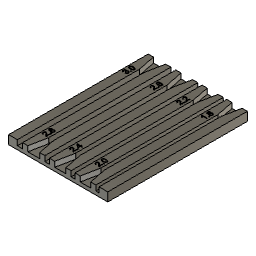
test_grooves (Autodesk Fusion 360 design; units mm, degrees)
Autodesk Fusion 360 part; units mm, degrees
sketch "Sketch1" plane through (0, 0, 0) normal (0, 0, 1) x (1, 0, 0)
  line L0 (0, 0) -> (56.8, 0)
  line L1 (56.8, 80) -> (0, 80)
  line L2 (0, 80) -> (0, 0)
  line L3 (0, 70) -> (117.6, 70) construction
  line L4 (5, 70) -> (5, 0)
  line L5 (8, 0) -> (8, 70)
  line L6 (5, 70) -> (3, 80)
  line L7 (8, 70) -> (10, 80)
  line L8 (20.8, 0) -> (20.8, 70)
  line L9 (23.4, 0) -> (23.4, 70)
  line L10 (35.8, 70) -> (35.8, 0)
  line L11 (38, 0) -> (38, 70)
  line L12 (18.8, 80) -> (20.8, 70)
  line L13 (25.4, 80) -> (23.4, 70)
  line L14 (50, 70) -> (50, 0)
  line L15 (51.8, 0) -> (51.8, 70)
  line L16 (35.8, 70) -> (33.8, 80)
  line L17 (38, 70) -> (40, 80)
  line L18 (50, 70) -> (48, 80)
  line L19 (51.8, 70) -> (53.8, 80)
  line L20 (56.8, 80) -> (56.8, 0)
  line L21 (0, 10) -> (56.8, 10) construction
  line L22 (13, 10) -> (13, 80)
  line L23 (15.8, 10) -> (15.8, 80)
  line L24 (13, 10) -> (11, 0)
  line L25 (15.8, 10) -> (17.8, 0)
  line L26 (28.4, 10) -> (28.4, 80)
  line L27 (30.8, 10) -> (30.8, 80)
  line L28 (43, 10) -> (43, 80)
  line L29 (45, 10) -> (45, 80)
  line L30 (28.4, 10) -> (26.4, 0)
  line L31 (30.8, 10) -> (32.8, 0)
  line L32 (43, 10) -> (41, 0)
  line L33 (45, 10) -> (47, 0)
  line L34 (4.6901, 63.9511) -> (4.6901, 69.9511) construction
  line L35 (4.6901, 69.9511) -> (0.6901, 69.9511) construction
  line L36 (0.6901, 69.9511) -> (0.6901, 63.9511) construction
  line L37 (0.6901, 63.9511) -> (4.6901, 63.9511) construction
  line L38 (12.2954, 9.9662) -> (12.3506, 15.4583) construction
  line L39 (12.3506, 15.4583) -> (8.7183, 15.4949) construction
  line L40 (8.7183, 15.4949) -> (8.6631, 10.0027) construction
  line L41 (8.6631, 10.0027) -> (12.2954, 9.9662) construction
  line L42 (27.6617, 10.1109) -> (27.6577, 16.1571) construction
  line L43 (27.6577, 16.1571) -> (24.105, 16.1548) construction
  line L44 (24.105, 16.1548) -> (24.109, 10.1086) construction
  line L45 (24.109, 10.1086) -> (27.6617, 10.1109) construction
  line L46 (35.0116, 64.0599) -> (35.0126, 69.9176) construction
  line L47 (35.0126, 69.9176) -> (31.4608, 69.9182) construction
  line L48 (31.4608, 69.9182) -> (31.4599, 64.0605) construction
  line L49 (31.4599, 64.0605) -> (35.0116, 64.0599) construction
  line L50 (42.3147, 10.1049) -> (42.3201, 16.1856) construction
  line L51 (42.3201, 16.1856) -> (38.7684, 16.1888) construction
  line L52 (38.7684, 16.1888) -> (38.763, 10.108) construction
  line L53 (38.763, 10.108) -> (42.3147, 10.1049) construction
  line L54 (49.2084, 64.0083) -> (49.2094, 69.8656) construction
  line L55 (49.2094, 69.8656) -> (45.6577, 69.8662) construction
  line L56 (45.6577, 69.8662) -> (45.6567, 64.0089) construction
  line L57 (45.6567, 64.0089) -> (49.2084, 64.0083) construction
  line L58 (20.0668, 63.882) -> (20.0677, 69.7397) construction
  line L59 (20.0677, 69.7397) -> (16.516, 69.7403) construction
  line L60 (16.516, 69.7403) -> (16.515, 63.8826) construction
  line L61 (16.515, 63.8826) -> (20.0668, 63.882) construction
  dimension "d1" = 80
  dimension "d2" = 70
  dimension "d3" = 3
  dimension "d4" = 2
  dimension "d5" = 2
  dimension "d6" = 5
  dimension "d11" = 2.6
  dimension "d17" = 2
  dimension "d18" = 2
  dimension "d20" = 2.2
  dimension "d25" = 2
  dimension "d26" = 2
  dimension "d28" = 1.8
  dimension "d33" = 2
  dimension "d34" = 2
  dimension "d35" = 5
  dimension "d50" = 70
  dimension "d51" = 2.8
  dimension "d52" = 2
  dimension "d53" = 2
  dimension "d54" = 5
  dimension "d55" = 5
  dimension "d56" = 5
  dimension "d57" = 2.4
  dimension "d58" = 2
  dimension "d59" = 2
  dimension "d60" = 5
  dimension "d61" = 2
  dimension "d62" = 5
  dimension "d67" = 3
  dimension "d68" = 3
  dimension "d70" = 3
  dimension "d71" = 3
  dimension "d72" = 3
  dimension "d73" = 3
  dimension "d74" = 3
  text T0 "3.0" font "Arial" height 3 align left top in box 6 x 4 at (4.6901, 63.9511) x (0, 1) y (-1, 0) spacing 1
  text T1 "2.8\n" font "Arial" height 3 align left top in box 5.4925 x 3.6325 at (12.2954, 9.9662) x (0.010065, 0.999949) y (-0.999949, 0.010065) spacing 1
  text T2 "2.4\n" font "Arial" height 3 align left top in box 6.0461 x 3.5527 at (27.6617, 10.1109) x (-0.000655, 1) y (-1, -0.000655) spacing 1
  text T3 "2.2" font "Arial" height 3 align left top in box 5.8577 x 3.5517 at (35.0116, 64.0599) x (0.000163, 1) y (-1, 0.000163) spacing 1
  text T4 "2.0" font "Arial" height 3 align left top in box 6.0807 x 3.5517 at (42.3147, 10.1049) x (0.000894, 1) y (-1, 0.000894) spacing 1
  text T5 "1.8\n" font "Arial" height 3 align left top in box 5.8573 x 3.5517 at (49.2084, 64.0083) x (0.000162, 1) y (-1, 0.000162) spacing 1
  text T6 "2.6\n" font "Arial" height 3 align left top in box 5.8577 x 3.5517 at (20.0668, 63.882) x (0.000163, 1) y (-1, 0.000163) spacing 1
  constraint horizontal L0
  constraint horizontal L1
  constraint vertical L2
  constraint coincident L0.start L2.end
  constraint coincident L2 L3.start
  constraint coincident L3 L4.start
  constraint coincident L0 L4.end
  constraint perpendicular L0 L4
  constraint coincident L0 L5.start
  constraint coincident L3 L5.end
  constraint perpendicular L3 L5
  constraint coincident L1 L6.end
  constraint coincident L1 L7.end
  constraint coincident L3 L10.start
  constraint coincident L0 L10.end
  constraint perpendicular L0 L10
  constraint coincident L0 L11.start
  constraint coincident L3 L11.end
  constraint perpendicular L3 L11
  constraint coincident L1 L12.start
  constraint coincident L1 L13.start
  constraint coincident L3 L8.end
  constraint coincident L3 L9.end
  constraint coincident L3 L14.start
  constraint coincident L0 L14.end
  constraint perpendicular L0 L14
  constraint coincident L0 L15.start
  constraint coincident L3 L15.end
  constraint perpendicular L3 L15
  constraint coincident L1 L17.end
  constraint coincident L1 L18.end
  constraint coincident L1 L19.end
  constraint perpendicular L0 L20
  constraint coincident L1 L16.end
  constraint coincident L2 L21.start
  constraint coincident L20 L21.end
  constraint perpendicular L20 L21
  constraint coincident L21 L22.start
  constraint coincident L1 L22.end
  constraint perpendicular L1 L22
  constraint coincident L21 L23.start
  constraint coincident L1 L23.end
  constraint perpendicular L1 L23
  constraint coincident L0 L24.end
  constraint coincident L0 L25.end
  constraint midpoint L21 L26.start
  constraint midpoint L1 L26.end
  constraint coincident L21 L27.start
  constraint coincident L1 L27.end
  constraint perpendicular L1 L27
  constraint coincident L21 L28.start
  constraint coincident L1 L28.end
  constraint perpendicular L1 L28
  constraint coincident L21 L29.start
  constraint coincident L1 L29.end
  constraint perpendicular L1 L29
  constraint coincident L0 L30.end
  constraint coincident L0 L31.end
  constraint coincident L0 L32.end
  constraint parallel L30 L32
  constraint coincident L0 L33.end
  constraint parallel L31 L33
  measures "d1" distance of L0 L1
  measures "d2" distance of L0 L3
  measures "d3" distance of L4 L5
  measures "d4" distance of L4 L6.end
  measures "d5" distance of L5 L7.end
  measures "d6" distance of L2 L4
  measures "d11" distance of L8 L9
  measures "d17" distance of L8 L12.start
  measures "d18" distance of L9 L13.start
  measures "d20" distance of L10 L11
  measures "d25" distance of L10 L16.end
  measures "d26" distance of L11 L17.end
  measures "d28" distance of L14 L15
  measures "d33" distance of L14 L18.end
  measures "d34" distance of L15 L19.end
  measures "d35" distance of L15 L20
  measures "d50" distance of L1 L21
  measures "d51" distance of L22 L23
  measures "d52" distance of L22 L24.end
  measures "d53" distance of L23 L25.end
  measures "d54" distance of L5 L22
  measures "d55" distance of L8 L23
  measures "d56" distance of L9 L26
  measures "d57" distance of L26 L27
  measures "d58" distance of L26 L30.end
  measures "d59" horizontal distance of L27.start L31.end
  measures "d60" distance of L10 L27
  measures "d61" distance of L28 L29
  measures "d62" distance of L11 L28
extrude "Extrude4" add sketch "Sketch1" against normal blind 5
extrude "Extrude5" cut sketch "Sketch1" against normal blind 3 contours L0 L1 L4 L5 L6 L7 | L0 L1 L22 L23 L24 L25 | L0 L1 L8 L9 L12 L13 | L0 L1 L26 L27 L30 L31 | L0 L1 L10 L11 L16 L17 | L0 L1 L28 L29 L32 L33 | L0 L1 L14 L15 L18 L19
extrude "Extrude6" cut sketch "Sketch1" against normal blind 1 text T6 T0 T1 T2 T3 T5 T4
equation "d5 = d4"
equation "d17 = d4"
equation "d18 = d4"
equation "d25 = d4"
equation "d26 = d4"
equation "d33 = d4"
equation "d34 = d4"
equation "d35 = d6"
equation "d52 = d4"
equation "d53 = d4"
equation "d54 = d6"
equation "d55 = d6"
equation "d56 = d6"
equation "d58 = d52"
equation "d59 = d52"
equation "d60 = d6"
equation "d62 = d6"
